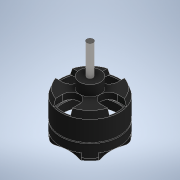
# Autodesk Inventor part: redox_bl_400_1400
Saved by Autodesk Inventor 2021 (Build 250183000, 183)
## iProperties
Created: 2022-05-14
Part Number: redox_bl_400_1400
Material: Generic
Document SubType Name: Modeling
Designer: ermoz
Density: 1 g/cm^3
Appearance: Default
Author: ermoz
Autodesk Inventor part; units mm, degrees
ref_plane "YZ Plane" through (0, 0, 0) normal (1, 0, 0) x (0, 1, 0)
ref_plane "XZ Plane" through (0, 0, 0) normal (0, 1, 0) x (-1, 0, 0)
ref_plane "XY Plane" through (0, 0, 0) normal (0, 0, 1) x (1, 0, 0)
sketch "Sketch1" plane through (0, 0, 0) normal (0, 1, 0) x (-1, 0, 0)
  circle A0 centre (0, 0) radius 14
  dimension "d0" = 28
  constraints: 1 centre point, 1 coincident
  measures "d0" diameter of A0
extrude "Extrusion1" add sketch "Sketch1" along normal blind 8
sketch "Sketch2" plane through (0, 8, 0) normal (0, 1, 0) x (1, 0, 0)
  circle A0 centre (0, 0) radius 1.5
  dimension "d3" = 3
  constraints: 1 centre point, 1 coincident
  measures "d3" diameter of A0
extrude "Extrusion2" cut sketch "Sketch2" against normal blind 8
extrude "Extrusion3" add sketch "Sketch2" along normal blind 32.5 and the other way blind 7 separate body
sketch "Sketch3" plane through (0, 0, 0) normal (0, -1, 0) x (1, 0, 0)
  circle A0 centre (0, 0) radius 3.75
  circle A1 centre (0, 0) radius 1.5
  dimension "d10" = 7.5
  constraints: 2 centre point, 2 coincident
  measures "d10" diameter of A0
extrude "Extrusion4" cut sketch "Sketch3" against normal through all contours A0 | A1 bodies 1
extrude "Extrusion5" add sketch "Sketch3" against normal blind 6 separate body
sketch "Sketch4" plane through (0, 0, 0) normal (0, -1, 0) x (1, 0, 0)
  circle A0 centre (0, 0) radius 3.75 projected
  circle A1 centre (0, 0) radius 1.5 projected
extrude "Extrusion6" cut sketch "Sketch4" against normal blind 2 bodies 3
sketch "Sketch5" plane through (0, 0, 0) normal (0, -1, 0) x (1, 0, 0)
  circle A0 centre (0, 0) radius 5
  dimension "d17" = 10
  constraints: 1 centre point, 1 coincident
  measures "d17" diameter of A0
extrude "Extrusion7" cut sketch "Sketch5" against normal blind 2 bodies 1
sketch "Sketch6" plane through (0, 2, 0) normal (0, -1, 0) x (1, 0, 0)
  circle A0 centre (0, 0) radius 2.125
  circle A1 centre (0, 0) radius 3.375
  dimension "d20" = 6.75
  dimension "d21" = 4.25
  constraints: 2 centre point, 2 coincident
  measures "d20" diameter of A1
  measures "d21" diameter of A0
extrude "Extrusion8" cut sketch "Sketch6" against normal blind 0.25 bodies 3
sketch "Sketch7" plane through (0, 8, 0) normal (0, 1, 0) x (1, 0, 0)
  circle A0 centre (0, 0) radius 14 projected
  circle A1 centre (0, 0) radius 13.2
  circle A2 centre (0, 0) radius 3.75 projected
  circle A3 centre (0, 0) radius 14
  dimension "d24" = 26.4
  constraints: 2 centre point, 2 coincident
  measures "d24" diameter of A1
extrude "Extrusion9" add sketch "Sketch7" along normal blind 13 contours A0 bodies 1
extrude "Extrusion10" cut sketch "Sketch7" along normal blind 0.5 contours A0 bodies 1
sketch "Sketch8" plane through (0, 21, 0) normal (0, 1, 0) x (1, 0, 0)
  circle A0 centre (0, 0) radius 14 projected
extrude "Extrusion11" add sketch "Sketch8" against normal blind 3 bodies 1
sketch "Sketch9" plane through (0, 21, 0) normal (0, 1, 0) x (1, 0, 0)
  circle A0 centre (0, 0) radius 5
  dimension "d31" = 10
  constraints: 1 centre point, 1 coincident
  measures "d31" diameter of A0
extrude "Extrusion12" add sketch "Sketch9" along normal blind 5 bodies 1
chamfer "Chamfer1" distance 1 distance2 3 1 edges at (-14, 21, 0) measured on face at (10.816, 21, 1.5157)
fillet "Fillet1" radius 2 1 edges at (14, 0, 0)
sketch "Sketch10" plane through (0, 0, 0) normal (0, -1, 0) x (1, 0, 0)
  circle A0 centre (0, 26) radius 16.25
  circle A1 centre (26, 0) radius 16.25
  circle A2 centre (0, -26) radius 16.25
  circle A3 centre (-26, 0) radius 16.25
  line L0 (0, 0) -> (17.3455, 0)
  circle A4 centre (0, 0) radius 1.5 projected
  line L1 (0, 0) -> (0, -21.6607)
  circle A5 centre (0, 0) radius 9.75
  dimension "d38" = 26
  dimension "d39" = 26
  dimension "d40" = 19.5
  constraints: 5 centre point, 4 end point, 3 equal radius, 2 point on line, 2 symmetric about line, 1 coincident, 1 horizontal, 1 tangent, 1 vertical, 1 vertical alignment
  measures "d38" distance of L0.start A2.centre
  measures "d39" distance of A1.centre L0.start
  measures "d40" diameter of A5
extrude "Extrusion13" cut sketch "Sketch10" against normal blind 4 contours A0 | A1 | A2 | A3 bodies 1
sketch "Sketch11" plane through (0, 8, 0) normal (0, 1, 0) x (1, 0, 0)
  circle A0 centre (0, 0) radius 13.2
  constraints: 1 centre point, 1 coincident
extrude "Extrusion14" cut sketch "Sketch11" against normal blind 5.5 bodies 1
fillet "Fillet2" radius 1.5 4 edges at (-9.3338, 2.5, -9.3338) (-9.3338, 2.5, 9.3338) (9.3338, 2.5, -9.3338) (9.3338, 2.5, 9.3338)
sketch "Sketch12" plane through (0, 21, 0) normal (0, 1, 0) x (1, 0, 0)
  circle A0 centre (9, 0) radius 4
  line L0 (35.4146, -4) -> (9, -4)
  line L1 (9, -4) -> (9, 4)
  line L2 (9, 4) -> (35.4146, 4)
  line L3 (35.4146, 4) -> (35.4146, -4)
  circle A1 centre (0, 0) radius 1.5 projected
  line L4 (0, 0) -> (40.9153, 0)
  circle A2 centre (0, 0) radius 5 projected
  circle A3 centre (0, -9) radius 4
  line L5 (-4, -35.4146) -> (-4, -9)
  line L6 (4, -9) -> (4, -35.4146)
  line L7 (-4, -9) -> (4, -9)
  line L8 (4, -35.4146) -> (-4, -35.4146)
  circle A4 centre (-9, 0) radius 4
  line L9 (-35.4146, 4) -> (-9, 4)
  line L10 (-9, -4) -> (-35.4146, -4)
  line L11 (-9, 4) -> (-9, -4)
  line L12 (-35.4146, -4) -> (-35.4146, 4)
  circle A5 centre (0, 9) radius 4
  line L13 (4, 35.4146) -> (4, 9)
  line L14 (-4, 9) -> (-4, 35.4146)
  line L15 (4, 9) -> (-4, 9)
  line L16 (-4, 35.4146) -> (4, 35.4146)
  dimension "d46" = 8
  dimension "d49" = 360
  constraints: 34 end point, 5 midpoint, 4 centre point, 3 tangent, 2 coincident, 2 horizontal, 2 parallel, 1 perpendicular, 1 point on line, 47 other
  measures "d46" diameter of A0
extrude "Extrusion15" cut sketch "Sketch12" against normal blind 3 contours L4 L1 A0 | L4 L3 L0 A0 | A0 L1 L4 | A0 L2 L3 L4 | L1 L4 A0 | A3 L7 | A4 L11 | A5 L15 | A0 L4 L1 | L14 L16 L13 A5 | A5 L15 | L6 L8 L5 A3 | A3 L7 | L11 A4 | A4 L10 L12 L9 bodies 1
sketch "Sketch13" plane through (0, 0, 0) normal (0, -1, 0) x (1, 0, 0)
  circle A0 centre (0, 0) radius 6.8
  line L0 (0, 0) -> (-8.9883, 8.9883)
  line L1 (0, 0) -> (12.7114, 0) construction
  circle A1 centre (-5.6922, 5.6922) radius 1.25
  circle A2 centre (-5.6922, -5.6922) radius 1.25
  circle A3 centre (5.6922, -5.6922) radius 1.25
  circle A4 centre (5.6922, 5.6922) radius 1.25
  dimension "d53" = 135
  dimension "d54" = 2.5
  dimension "d55" = 13.6
  dimension "d58" = 360
  constraints: 5 centre point, 4 end point, 1 coincident, 1 equal length, 1 horizontal, 1 point on line, 1 tangent, 9 other
  measures "d53" angle of L1 L0
  measures "d54" diameter of A1
  measures "d55" diameter of A0
extrude "Extrusion16" cut sketch "Sketch13" against normal blind 3 contours A3 | A2 | A1 L0 | L0 A1 | A4 bodies 1
thread "Thread1" size "M2.5x0.45" class "6H" standard "ANSI Metric M Profile" full length
thread "Thread2" size "M2.5x0.45" class "6H" standard "ANSI Metric M Profile" full length
thread "Thread3" size "M2.5x0.45" class "6H" standard "ANSI Metric M Profile" full length
thread "Thread4" size "M2.5x0.45" class "6H" standard "ANSI Metric M Profile" full length
equation "\"d39\" = d38"
body "Solid1"
body "Solid2"
body "Solid3"
